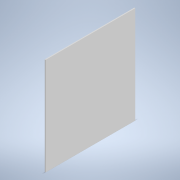
# Autodesk Inventor part: Front_left
Saved by Autodesk Inventor 2020 (Build 240168000, 168)
## iProperties
Created: 2020-08-08
Part Number: Front_left
Material: Generic
Document SubType Name: Modeling
Designer: Abbas
Density: 1 g/cm^3
Appearance: Default
Author: Abbas
Autodesk Inventor part; units mm, degrees
ref_plane "YZ Plane" through (0, 0, 0) normal (1, 0, 0) x (0, 1, 0)
ref_plane "XZ Plane" through (0, 0, 0) normal (0, 1, 0) x (-1, 0, 0)
ref_plane "XY Plane" through (0, 0, 0) normal (0, 0, 1) x (1, 0, 0)
sketch "Sketch1" plane through (0, 0, 0) normal (1, 0, 0) x (0, 1, 0)
  line L0 (156, 143.5) -> (-156, 143.5)
  line L1 (-156, 143.5) -> (-156, -143.5)
  line L2 (-156, -143.5) -> (156, -143.5)
  line L3 (156, -143.5) -> (156, 143.5)
  line L4 (156, 143.5) -> (-156, -143.5) construction
  line L5 (-156, 143.5) -> (156, -143.5) construction
  point P0 (0, 0)
  dimension "d0" = 312
  dimension "d1" = 287
  constraints: 12 end point, 2 midpoint, 2 parallel, 1 horizontal, 1 perpendicular
  measures "d0" distance of L2.end L1.end
  measures "d1" distance of L1.end L0.end
extrude "Extrusion1" add sketch "Sketch1" along normal blind 3
body "Solid1"
